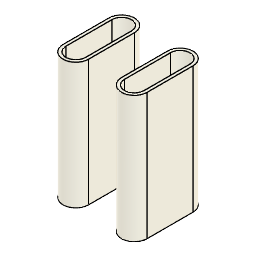
shuffle-cover (Autodesk Fusion 360 design; units mm, degrees)
Autodesk Fusion 360 part; units mm, degrees
sketch "shuffle-cover" plane through (0, 0, 0) normal (0, 0, 1) x (1, 0, 0)
  circle A0 centre (-0.0001, 7.5921) radius 1.1 construction
  line L0 (-3.2401, 2.9921) -> (3.2399, 2.9921) construction
  line L1 (-2.7401, -7.6079) -> (-2.7401, 7.5921)
  arc A1 (3.2399, 7.5921) -> (-3.2401, 7.5921) centre (-0.0001, 7.5921) ccw
  line L2 (3.2399, -7.6079) -> (3.2399, 7.5921)
  arc A2 (-2.7401, -7.6079) -> (2.7399, -7.6079) centre (-0.0001, -7.6079) ccw
  circle A3 centre (-0.0001, -0.0079) radius 1.7 construction
  arc A4 (-3.2401, -7.6079) -> (3.2399, -7.6079) centre (-0.0001, -7.6079) ccw
  circle A5 centre (-0.0001, 7.5921) radius 1.9 construction
  line L3 (2.7399, -7.6079) -> (2.7399, 7.5921)
  line L4 (-3.2401, -7.6079) -> (-3.2401, 7.5921)
  arc A6 (2.7399, 7.5921) -> (-2.7401, 7.5921) centre (-0.0001, 7.5921) ccw
  circle A7 centre (-0.0001, -7.6079) radius 1.9 construction
  circle A8 centre (-0.0001, -7.6079) radius 1.1 construction
  circle A9 centre (-0.0001, -0.0079) radius 1.3 construction
  line L5 (-3.2401, -3.0079) -> (3.2399, -3.0079) construction
  line L6 (-23.64, -7.6) -> (-23.64, 7.6)
  circle A10 centre (-19.4, -7.6) radius 1.9
  arc A11 (-15.16, 7.6) -> (-23.64, 7.6) centre (-19.4, 7.6) ccw
  circle A12 centre (-19.4, 7.6) radius 1.1
  line L7 (-22.64, -3) -> (-16.16, -3)
  arc A13 (-23.64, -7.6) -> (-15.16, -7.6) centre (-19.4, -7.6) ccw
  arc A14 (-16.16, 7.6) -> (-22.64, 7.6) centre (-19.4, 7.6) ccw
  line L8 (-22.64, -7.6) -> (-22.64, 7.6)
  arc A15 (-22.64, -7.6) -> (-16.16, -7.6) centre (-19.4, -7.6) ccw
  circle A16 centre (-19.4, 0) radius 1.3
  circle A17 centre (-19.4, 0) radius 1.7
  line L9 (-16.16, -7.6) -> (-16.16, 7.6)
  circle A18 centre (-19.4, 7.6) radius 1.9
  line L10 (-15.16, -7.6) -> (-15.16, 7.6)
  circle A19 centre (-19.4, -7.6) radius 1.1
  line L11 (-22.64, 3) -> (-16.16, 3)
  arc A20 (4.2399, 7.5921) -> (-4.2401, 7.5921) centre (-0.0001, 7.5921) ccw
  line L12 (-4.2401, -7.6079) -> (-4.2401, 7.5921)
  arc A21 (-4.2401, -7.6079) -> (4.2399, -7.6079) centre (-0.0001, -7.6079) ccw
  line L13 (4.2399, -7.6079) -> (4.2399, 7.5921)
  point P0 (-0.0001, -0.0079)
  point P1 (-0.0001, -0.0079)
  point P2 (-19.4, 0)
  point P3 (-19.4, 0)
  dimension "d1" = 2.6
  dimension "d2" = 3.8
  dimension "d3" = 2.2
  dimension "d4" = 3.8
  dimension "d5" = 2.2
  dimension "d6" = 3.4
  dimension "d7" = 2.6
  dimension "d8" = 3.8
  dimension "d9" = 2.2
  dimension "d10" = 3.8
  dimension "d11" = 2.2
  dimension "d12" = 3.4
  constraint coincident P1 P0
  constraint concentric A7 A8
  constraint concentric A0 A5
  constraint concentric A3 A9
  constraint coincident L0.end L2
  constraint coincident L5.end L2
  constraint coincident L0.start L4
  constraint coincident L5.start L4
  constraint concentric A1 A6
  constraint concentric A2 A4
  constraint coincident P3 P2
  constraint concentric A10 A19
  constraint concentric A12 A18
  constraint concentric A16 A17
  constraint concentric A11 A14
  constraint concentric A13 A15
  constraint coincident L11.end L9
  constraint perpendicular L9 L11
  constraint coincident L7.end L9
  constraint perpendicular L7 L9
  constraint coincident L11.start L8
  constraint coincident L7.start L8
  constraint concentric A1 A20
  constraint concentric A4 A21
  measures "d1" diameter of A9
  measures "d2" diameter of A7
  measures "d3" diameter of A8
  measures "d4" diameter of A5
  measures "d5" diameter of A0
  measures "d6" diameter of A3
  measures "d7" diameter of A16
  measures "d8" diameter of A10
  measures "d9" diameter of A19
  measures "d10" diameter of A18
  measures "d11" diameter of A12
  measures "d12" diameter of A17
extrude "Extrude36" add sketch "shuffle-cover" along normal blind 2 contours A10 | L7 L8 A15 L9 | A14 L8 L9 L11 | A18 makes body 1 at (-19.4274, -4.1677, 0) makes body 2 at (-19.3726, 4.1677, 0)
extrude "Extrude37" add sketch "shuffle-cover" along normal blind 1.6 contours L7 L8 L9 L11 | A17 bodies 1 2
extrude "Extrude38" add sketch "shuffle-cover" along normal blind 41.8 contours L6 A11 A13 L10 bodies 1
extrude "Extrude39" cut sketch "shuffle-cover" along normal blind 0.3 contours A10 | A17 | A18 bodies 1
chamfer "Chamfer19" distance 0.8 angle 45 2 edges at (-19.7978, -8.6256, 0.3) (-19.7978, 6.5744, 0.3) measured on face at (-18.3055, -7.7095, 0.8667) measured on face at (-19.6979, 8.6589, 0.8667) on bodies 1
chamfer "Chamfer20" distance 0.4 angle 45 1 edges at (-19.8701, -1.212, 0.3) measured on face at (-18.1065, -0.1294, 0.7333) on bodies 1
extrude "Extrude40" add sketch "shuffle-cover" along normal blind 1 from surface at 1.2 separate body contours A1 L2 A4 L4 makes body 3
chamfer "Chamfer21" distance 0.5 angle 45 4 edges at (-2.7401, -0.0079, 1.2) (-0.0001, 10.3321, 1.2) (2.7399, -0.0079, 1.2) (-0.0001, -10.3479, 1.2) measured on face at (-2.7401, -2.5412, 1.5333) measured on face at (-2.7367, 7.7287, 1.8667) measured on face at (2.7399, 2.5254, 1.8667) measured on face at (2.5746, -8.545, 1.8667) on bodies 3
extrude "Extrude41" add sketch "shuffle-cover" along normal blind 42 contours A20 L12 A21 L13 bodies 3
named bodies: "shuffle-cover-v1", "shuffle-cover-v2"
